Autodesk Inventor part; units mm, degrees
(part 2 of 2)
sketch "Sketch4" plane through (0, 2.3813, 0) normal (0, 1, 0) x (1, 0, 0)
  line L0 (28.188, 43.6739) -> (29.5096, 45.2433) construction
  spline S0 degree 3 poles (28.188, 43.6739) (29.5096, 45.2433) (31.9877, 45.6564) (33.3919, 45.6563) (35.0439, 45.6563) (37.3568, 44.8303) (37.3568, 41.6915) (37.3568, 40.122) (36.8611, 38.3874) (35.8699, 37.3136) knots 15 15 15 15 16 16 16 17 17 17 18 18 18 18
  line L1 (29.5096, 45.2433) -> (31.9877, 45.6564) construction
  line L2 (31.9877, 45.6564) -> (33.3919, 45.6563) construction
  line L3 (33.3919, 45.6563) -> (35.0439, 45.6563) construction
  line L4 (35.0439, 45.6563) -> (37.3568, 44.8303) construction
  line L5 (37.3568, 44.8303) -> (37.3568, 41.6915) construction
  line L6 (37.3568, 41.6915) -> (37.3568, 40.122) construction
  line L7 (37.3568, 40.122) -> (36.8611, 38.3874) construction
  line L8 (36.8611, 38.3874) -> (35.8699, 37.3136) construction
  spline S1 degree 3 poles (35.8699, 37.3136) (34.7135, 35.9094) (33.6397, 35.8268) (31.8224, 35.6616) (30.9138, 35.579) (30.8312, 35.579) (30.666, 35.579) (30.5834, 35.579) (30.253, 35.4964) (30.253, 35.0833) knots 18 18 18 18 19 19 19 20 20 20 21 21 21 21
  line L9 (35.8699, 37.3136) -> (34.7135, 35.9094) construction
  line L10 (34.7135, 35.9094) -> (33.6397, 35.8268) construction
  line L11 (33.6397, 35.8268) -> (31.8224, 35.6616) construction
  line L12 (31.8224, 35.6616) -> (30.9138, 35.579) construction
  line L13 (30.9138, 35.579) -> (30.8312, 35.579) construction
  line L14 (30.8312, 35.579) -> (30.666, 35.579) construction
  line L15 (30.666, 35.579) -> (30.5834, 35.579) construction
  line L16 (30.5834, 35.579) -> (30.253, 35.4964) construction
  line L17 (30.253, 35.4964) -> (30.253, 35.0833) construction
  spline S2 degree 3 poles (30.253, 35.0833) (30.253, 34.5877) (30.5834, 34.5877) (31.2442, 34.5877) knots 21 21 21 21 22 22 22 22
  line L18 (30.253, 35.0833) -> (30.253, 34.5877) construction
  line L19 (30.253, 34.5877) -> (30.5834, 34.5877) construction
  line L20 (30.5834, 34.5877) -> (31.2442, 34.5877) construction
  line L21 (31.2442, 34.5877) -> (33.2267, 34.5877)
  line L22 (13.0236, 12.4263) -> (20.0234, 12.4263)
  spline S3 degree 3 poles (20.0234, 12.4263) (20.3837, 12.4263) (20.8984, 12.4263) (20.8984, 12.9925) knots 1 1 1 1 2 2 2 2
  line L23 (20.0234, 12.4263) -> (20.3837, 12.4263) construction
  line L24 (20.3837, 12.4263) -> (20.8984, 12.4263) construction
  line L25 (20.8984, 12.4263) -> (20.8984, 12.9925) construction
  spline S4 degree 3 poles (20.8984, 12.9925) (20.8984, 13.5587) (20.3837, 13.5587) (20.0234, 13.5587) knots 2 2 2 2 3 3 3 3
  line L26 (20.8984, 12.9925) -> (20.8984, 13.5587) construction
  line L27 (20.8984, 13.5587) -> (20.3837, 13.5587) construction
  line L28 (20.3837, 13.5587) -> (20.0234, 13.5587) construction
  line L29 (20.0234, 13.5587) -> (13.0236, 13.5587)
  line L30 (13.0236, 13.5587) -> (13.0236, 20.4555)
  spline S5 degree 3 poles (13.0236, 20.4555) (13.0236, 20.8673) (13.0236, 21.4334) (12.4574, 21.4334) (11.8913, 21.4334) (11.8913, 20.9187) (11.8913, 20.5585) knots 5 5 5 5 6 6 6 7 7 7 7
  line L31 (13.0236, 20.4555) -> (13.0236, 20.8673) construction
  line L32 (13.0236, 20.8673) -> (13.0236, 21.4334) construction
  line L33 (13.0236, 21.4334) -> (12.4574, 21.4334) construction
  line L34 (12.4574, 21.4334) -> (11.8913, 21.4334) construction
  line L35 (11.8913, 21.4334) -> (11.8913, 20.9187) construction
  line L36 (11.8913, 20.9187) -> (11.8913, 20.5585) construction
  line L37 (11.8913, 20.5585) -> (11.8913, 13.5587)
  line L38 (11.8913, 13.5587) -> (4.8915, 13.5587)
  spline S6 degree 3 poles (4.8915, 13.5587) (4.5312, 13.5587) (3.965, 13.5587) (3.965, 12.9925) knots 9 9 9 9 10 10 10 10
  line L39 (4.8915, 13.5587) -> (4.5312, 13.5587) construction
  line L40 (4.5312, 13.5587) -> (3.965, 13.5587) construction
  line L41 (3.965, 13.5587) -> (3.965, 12.9925) construction
  spline S7 degree 3 poles (3.965, 12.9925) (3.965, 12.4264) (4.5312, 12.4264) (4.8915, 12.4263) knots 10 10 10 10 11 11 11 11
  line L42 (3.965, 12.9925) -> (3.965, 12.4264) construction
  line L43 (3.965, 12.4264) -> (4.5312, 12.4264) construction
  line L44 (4.5312, 12.4264) -> (4.8915, 12.4263) construction
  line L45 (4.8915, 12.4263) -> (11.8913, 12.4263)
  line L46 (11.8913, 12.4263) -> (11.8913, 5.6324)
  line L47 (11.8913, 5.6324) -> (4.8915, 5.6324)
  spline S8 degree 3 poles (4.8915, 5.6324) (4.5312, 5.6324) (3.965, 5.6324) (3.965, 5.0663) knots 14 14 14 14 15 15 15 15
  line L48 (4.8915, 5.6324) -> (4.5312, 5.6324) construction
  line L49 (4.5312, 5.6324) -> (3.965, 5.6324) construction
  line L50 (3.965, 5.6324) -> (3.965, 5.0663) construction
  spline S9 degree 3 poles (3.965, 5.0663) (3.965, 4.5001) (4.5312, 4.5001) (4.8915, 4.5001) knots 15 15 15 15 16 16 16 16
  line L51 (3.965, 5.0663) -> (3.965, 4.5001) construction
  line L52 (3.965, 4.5001) -> (4.5312, 4.5001) construction
  line L53 (4.5312, 4.5001) -> (4.8915, 4.5001) construction
  line L54 (4.8915, 4.5001) -> (20.0234, 4.5001)
  spline S10 degree 3 poles (20.0234, 4.5001) (20.3837, 4.5001) (20.8984, 4.5001) (20.8984, 5.0663) knots 17 17 17 17 18 18 18 18
  line L55 (20.0234, 4.5001) -> (20.3837, 4.5001) construction
  line L56 (20.3837, 4.5001) -> (20.8984, 4.5001) construction
  line L57 (20.8984, 4.5001) -> (20.8984, 5.0663) construction
  spline S11 degree 3 poles (20.8984, 5.0663) (20.8984, 5.6324) (20.3837, 5.6324) (20.0234, 5.6324) knots 18 18 18 18 19 19 19 19
  line L58 (20.8984, 5.0663) -> (20.8984, 5.6324) construction
  line L59 (20.8984, 5.6324) -> (20.3837, 5.6324) construction
  line L60 (20.3837, 5.6324) -> (20.0234, 5.6324) construction
  line L61 (20.0234, 5.6324) -> (13.0236, 5.6324)
  line L62 (13.0236, 5.6324) -> (13.0236, 12.4263)
  spline S12 degree 3 poles (33.2267, 34.5877) (36.1177, 34.5877) (38.1828, 32.6053) (38.1828, 28.6404) (38.1828, 24.0973) (35.4569, 22.6931) (33.3919, 22.6931) (31.905, 22.6931) (28.601, 23.1061) (27.1141, 25.3364) knots 0 0 0 0 1 1 1 2 2 2 3 3 3 3
  line L63 (33.2267, 34.5877) -> (36.1177, 34.5877) construction
  line L64 (36.1177, 34.5877) -> (38.1828, 32.6053) construction
  line L65 (38.1828, 32.6053) -> (38.1828, 28.6404) construction
  line L66 (38.1828, 28.6404) -> (38.1828, 24.0973) construction
  line L67 (38.1828, 24.0973) -> (35.4569, 22.6931) construction
  line L68 (35.4569, 22.6931) -> (33.3919, 22.6931) construction
  line L69 (33.3919, 22.6931) -> (31.905, 22.6931) construction
  line L70 (31.905, 22.6931) -> (28.601, 23.1061) construction
  line L71 (28.601, 23.1061) -> (27.1141, 25.3364) construction
  spline S13 degree 3 poles (27.1141, 25.3364) (28.8488, 25.3364) (29.2618, 26.5754) (29.2618, 27.4014) (29.2618, 28.5578) (28.3532, 29.3838) (27.1968, 29.3838) (26.2055, 29.3838) (25.1317, 28.723) (25.1317, 27.2362) (25.1317, 23.7669) (28.9314, 21.5367) (33.3919, 21.5367) (38.5132, 21.5367) (42.065, 25.0059) (42.065, 28.6404) (42.065, 31.5315) (39.7522, 34.4225) (35.7047, 35.2485) knots 3 3 3 3 4 4 4 5 5 5 6 6 6 7 7 7 8 8 8 9 9 9 9
  line L72 (27.1141, 25.3364) -> (28.8488, 25.3364) construction
  line L73 (28.8488, 25.3364) -> (29.2618, 26.5754) construction
  line L74 (29.2618, 26.5754) -> (29.2618, 27.4014) construction
  line L75 (29.2618, 27.4014) -> (29.2618, 28.5578) construction
  line L76 (29.2618, 28.5578) -> (28.3532, 29.3838) construction
  line L77 (28.3532, 29.3838) -> (27.1968, 29.3838) construction
  line L78 (27.1968, 29.3838) -> (26.2055, 29.3838) construction
  line L79 (26.2055, 29.3838) -> (25.1317, 28.723) construction
  line L80 (25.1317, 28.723) -> (25.1317, 27.2362) construction
  line L81 (25.1317, 27.2362) -> (25.1317, 23.7669) construction
  line L82 (25.1317, 23.7669) -> (28.9314, 21.5367) construction
  line L83 (28.9314, 21.5367) -> (33.3919, 21.5367) construction
  line L84 (33.3919, 21.5367) -> (38.5132, 21.5367) construction
  line L85 (38.5132, 21.5367) -> (42.065, 25.0059) construction
  line L86 (42.065, 25.0059) -> (42.065, 28.6404) construction
  line L87 (42.065, 28.6404) -> (42.065, 31.5315) construction
  line L88 (42.065, 31.5315) -> (39.7522, 34.4225) construction
  line L89 (39.7522, 34.4225) -> (35.7047, 35.2485) construction
  spline S14 degree 3 poles (35.7047, 35.2485) (39.5044, 36.6528) (40.9086, 39.3786) (40.9086, 41.6915) (40.9086, 44.5825) (37.6046, 46.7302) (33.4745, 46.7302) (29.427, 46.7302) (26.2881, 44.7477) (26.2881, 41.7741) (26.2881, 40.5351) (27.1142, 39.8742) (28.188, 39.8742) (29.3444, 39.8742) (30.0878, 40.7003) (30.0878, 41.6915) (30.0878, 42.7653) (29.3444, 43.5913) (28.188, 43.6739) knots 9 9 9 9 10 10 10 11 11 11 12 12 12 13 13 13 14 14 14 15 15 15 15
  line L90 (35.7047, 35.2485) -> (39.5044, 36.6528) construction
  line L91 (39.5044, 36.6528) -> (40.9086, 39.3786) construction
  line L92 (40.9086, 39.3786) -> (40.9086, 41.6915) construction
  line L93 (40.9086, 41.6915) -> (40.9086, 44.5825) construction
  line L94 (40.9086, 44.5825) -> (37.6046, 46.7302) construction
  line L95 (37.6046, 46.7302) -> (33.4745, 46.7302) construction
  line L96 (33.4745, 46.7302) -> (29.427, 46.7302) construction
  line L97 (29.427, 46.7302) -> (26.2881, 44.7477) construction
  line L98 (26.2881, 44.7477) -> (26.2881, 41.7741) construction
  line L99 (26.2881, 41.7741) -> (26.2881, 40.5351) construction
  line L100 (26.2881, 40.5351) -> (27.1142, 39.8742) construction
  line L101 (27.1142, 39.8742) -> (28.188, 39.8742) construction
  line L102 (28.188, 39.8742) -> (29.3444, 39.8742) construction
  line L103 (29.3444, 39.8742) -> (30.0878, 40.7003) construction
  line L104 (30.0878, 40.7003) -> (30.0878, 41.6915) construction
  line L105 (30.0878, 41.6915) -> (30.0878, 42.7653) construction
  line L106 (30.0878, 42.7653) -> (29.3444, 43.5913) construction
  line L107 (29.3444, 43.5913) -> (28.188, 43.6739) construction
  line L108 (25.1359, -42.0708) -> (-42.6059, -42.0708)
  line L109 (-42.6059, -42.0708) -> (-42.6059, 25.671)
  line L110 (-42.6059, 25.671) -> (17.5159, 25.671)
  spline S15 degree 3 poles (17.5159, 25.671) (20.4794, 22.7075) (22.1725, 21.0145) (25.1359, 18.051) knots 3 3 3 3 4 4 4 4
  line L111 (17.5159, 25.671) -> (20.4794, 22.7075) construction
  line L112 (20.4794, 22.7075) -> (22.1725, 21.0145) construction
  line L113 (22.1725, 21.0145) -> (25.1359, 18.051) construction
  line L114 (25.1359, 18.051) -> (25.1359, -42.0708)
  spline S16 degree 3 poles (-17.3729, 2.4446) (-16.9814, 3.7171) (-16.3941, 6.1641) (-16.3941, 6.4577) knots 0 0 0 0 1 1 1 1
  line L115 (-17.3729, 2.4446) -> (-16.9814, 3.7171) construction
  line L116 (-16.9814, 3.7171) -> (-16.3941, 6.1641) construction
  line L117 (-16.3941, 6.1641) -> (-16.3941, 6.4577) construction
  spline S17 degree 3 poles (-16.3941, 6.4577) (-16.3941, 7.5344) (-17.1772, 8.1217) (-18.2539, 8.1217) knots 1 1 1 1 2 2 2 2
  line L118 (-16.3941, 6.4577) -> (-16.3941, 7.5344) construction
  line L119 (-16.3941, 7.5344) -> (-17.1772, 8.1217) construction
  line L120 (-17.1772, 8.1217) -> (-18.2539, 8.1217) construction
  spline S18 degree 3 poles (-18.2539, 8.1217) (-18.3517, 8.1217) (-20.1136, 8.0238) (-20.7009, 5.8705) knots 2 2 2 2 3 3 3 3
  line L121 (-18.2539, 8.1217) -> (-18.3517, 8.1217) construction
  line L122 (-18.3517, 8.1217) -> (-20.1136, 8.0238) construction
  line L123 (-20.1136, 8.0238) -> (-20.7009, 5.8705) construction
  line L124 (-20.7009, 5.8705) -> (-29.7059, -30.2475)
  spline S19 degree 3 poles (-29.7059, -30.2475) (-29.9017, -31.0305) (-29.9017, -31.1284) (-29.9017, -31.3241) knots 4 4 4 4 5 5 5 5
  line L125 (-29.7059, -30.2475) -> (-29.9017, -31.0305) construction
  line L126 (-29.9017, -31.0305) -> (-29.9017, -31.1284) construction
  line L127 (-29.9017, -31.1284) -> (-29.9017, -31.3241) construction
  spline S20 degree 3 poles (-29.9017, -31.3241) (-29.9017, -32.2051) (-29.2165, -32.9881) (-28.1398, -32.9881) (-26.8674, -32.9881) (-26.0843, -31.8136) (-25.9864, -31.6178) knots 5 5 5 5 6 6 6 7 7 7 7
  line L128 (-29.9017, -31.3241) -> (-29.9017, -32.2051) construction
  line L129 (-29.9017, -32.2051) -> (-29.2165, -32.9881) construction
  line L130 (-29.2165, -32.9881) -> (-28.1398, -32.9881) construction
  line L131 (-28.1398, -32.9881) -> (-26.8674, -32.9881) construction
  line L132 (-26.8674, -32.9881) -> (-26.0843, -31.8136) construction
  line L133 (-26.0843, -31.8136) -> (-25.9864, -31.6178) construction
  spline S21 degree 3 poles (-25.9864, -31.6178) (-25.6928, -31.1284) (-24.9098, -27.8004) (-22.5606, -18.2082) knots 7 7 7 7 8 8 8 8
  line L134 (-25.9864, -31.6178) -> (-25.6928, -31.1284) construction
  line L135 (-25.6928, -31.1284) -> (-24.9098, -27.8004) construction
  line L136 (-24.9098, -27.8004) -> (-22.5606, -18.2082) construction
  spline S22 degree 3 poles (-22.5606, -18.2082) (-20.5051, -19.8721) (-17.6666, -20.1658) (-16.492, -20.1658) (-12.0874, -20.1658) (-9.6404, -17.3272) (-8.1722, -15.5654) knots 8 8 8 8 9 9 9 10 10 10 10
  line L137 (-22.5606, -18.2082) -> (-20.5051, -19.8721) construction
  line L138 (-20.5051, -19.8721) -> (-17.6666, -20.1658) construction
  line L139 (-17.6666, -20.1658) -> (-16.492, -20.1658) construction
  line L140 (-16.492, -20.1658) -> (-12.0874, -20.1658) construction
  line L141 (-12.0874, -20.1658) -> (-9.6404, -17.3272) construction
  line L142 (-9.6404, -17.3272) -> (-8.1722, -15.5654) construction
  spline S23 degree 3 poles (-8.1722, -15.5654) (-7.5849, -18.4039) (-5.2358, -20.1658) (-2.4951, -20.1658) (-0.3417, -20.1658) (1.1265, -18.6976) (2.1053, -16.74) knots 10 10 10 10 11 11 11 12 12 12 12
  line L143 (-8.1722, -15.5654) -> (-7.5849, -18.4039) construction
  line L144 (-7.5849, -18.4039) -> (-5.2358, -20.1658) construction
  line L145 (-5.2358, -20.1658) -> (-2.4951, -20.1658) construction
  line L146 (-2.4951, -20.1658) -> (-0.3417, -20.1658) construction
  line L147 (-0.3417, -20.1658) -> (1.1265, -18.6976) construction
  line L148 (1.1265, -18.6976) -> (2.1053, -16.74) construction
  spline S24 degree 3 poles (2.1053, -16.74) (3.182, -14.4887) (3.965, -10.6714) (3.965, -10.5735) knots 12 12 12 12 13 13 13 13
  line L149 (2.1053, -16.74) -> (3.182, -14.4887) construction
  line L150 (3.182, -14.4887) -> (3.965, -10.6714) construction
  line L151 (3.965, -10.6714) -> (3.965, -10.5735) construction
  spline S25 degree 3 poles (3.965, -10.5735) (3.965, -9.8883) (3.3777, -9.8883) (3.182, -9.8883) (2.5947, -9.8883) (2.4968, -10.182) (2.301, -11.0629) knots 13 13 13 13 14 14 14 15 15 15 15
  line L152 (3.965, -10.5735) -> (3.965, -9.8883) construction
  line L153 (3.965, -9.8883) -> (3.3777, -9.8883) construction
  line L154 (3.3777, -9.8883) -> (3.182, -9.8883) construction
  line L155 (3.182, -9.8883) -> (2.5947, -9.8883) construction
  line L156 (2.5947, -9.8883) -> (2.4968, -10.182) construction
  line L157 (2.4968, -10.182) -> (2.301, -11.0629) construction
  spline S26 degree 3 poles (2.301, -11.0629) (1.3222, -15.076) (0.1477, -18.7955) (-2.3972, -18.7955) (-4.0612, -18.7955) (-4.257, -17.1315) (-4.257, -15.9569) (-4.257, -14.5866) (-3.5718, -11.6502) (-3.0824, -9.3989) knots 15 15 15 15 16 16 16 17 17 17 18 18 18 18
  line L158 (2.301, -11.0629) -> (1.3222, -15.076) construction
  line L159 (1.3222, -15.076) -> (0.1477, -18.7955) construction
  line L160 (0.1477, -18.7955) -> (-2.3972, -18.7955) construction
  line L161 (-2.3972, -18.7955) -> (-4.0612, -18.7955) construction
  line L162 (-4.0612, -18.7955) -> (-4.257, -17.1315) construction
  line L163 (-4.257, -17.1315) -> (-4.257, -15.9569) construction
  line L164 (-4.257, -15.9569) -> (-4.257, -14.5866) construction
  line L165 (-4.257, -14.5866) -> (-3.5718, -11.6502) construction
  line L166 (-3.5718, -11.6502) -> (-3.0824, -9.3989) construction
  line L167 (-3.0824, -9.3989) -> (-1.3205, -2.6452)
  spline S27 degree 3 poles (-1.3205, -2.6452) (-1.1248, -1.7642) (-0.4396, 0.5849) (-0.2438, 1.5637) (0.0498, 3.0319) (0.735, 5.381) (0.735, 5.7726) knots 19 19 19 19 20 20 20 21 21 21 21
  line L168 (-1.3205, -2.6452) -> (-1.1248, -1.7642) construction
  line L169 (-1.1248, -1.7642) -> (-0.4396, 0.5849) construction
  line L170 (-0.4396, 0.5849) -> (-0.2438, 1.5637) construction
  line L171 (-0.2438, 1.5637) -> (0.0498, 3.0319) construction
  line L172 (0.0498, 3.0319) -> (0.735, 5.381) construction
  line L173 (0.735, 5.381) -> (0.735, 5.7726) construction
  spline S28 degree 3 poles (0.735, 5.7726) (0.735, 6.8492) (-0.146, 7.4365) (-1.1248, 7.4365) (-1.4184, 7.4365) (-3.0824, 7.3386) (-3.5718, 5.2832) knots 21 21 21 21 22 22 22 23 23 23 23
  line L174 (0.735, 5.7726) -> (0.735, 6.8492) construction
  line L175 (0.735, 6.8492) -> (-0.146, 7.4365) construction
  line L176 (-0.146, 7.4365) -> (-1.1248, 7.4365) construction
  line L177 (-1.1248, 7.4365) -> (-1.4184, 7.4365) construction
  line L178 (-1.4184, 7.4365) -> (-3.0824, 7.3386) construction
  line L179 (-3.0824, 7.3386) -> (-3.5718, 5.2832) construction
  line L180 (-3.5718, 5.2832) -> (-6.5082, -6.4625)
  spline S29 degree 3 poles (-6.5082, -6.4625) (-7.1934, -9.5947) (-7.8785, -12.1396) (-8.0743, -12.8247) knots 24 24 24 24 25 25 25 25
  line L181 (-6.5082, -6.4625) -> (-7.1934, -9.5947) construction
  line L182 (-7.1934, -9.5947) -> (-7.8785, -12.1396) construction
  line L183 (-7.8785, -12.1396) -> (-8.0743, -12.8247) construction
  spline S30 degree 3 poles (-8.0743, -12.8247) (-8.1722, -13.1184) (-11.1086, -18.7954) (-16.1984, -18.7954) (-19.3306, -18.7954) (-20.7988, -16.74) (-20.7988, -13.3141) (-20.7988, -11.5523) (-20.4072, -9.7904) (-19.9178, -8.0286) knots 25 25 25 25 26 26 26 27 27 27 28 28 28 28
  line L184 (-8.0743, -12.8247) -> (-8.1722, -13.1184) construction
  line L185 (-8.1722, -13.1184) -> (-11.1086, -18.7954) construction
  line L186 (-11.1086, -18.7954) -> (-16.1984, -18.7954) construction
  line L187 (-16.1984, -18.7954) -> (-19.3306, -18.7954) construction
  line L188 (-19.3306, -18.7954) -> (-20.7988, -16.74) construction
  line L189 (-20.7988, -16.74) -> (-20.7988, -13.3141) construction
  line L190 (-20.7988, -13.3141) -> (-20.7988, -11.5523) construction
  line L191 (-20.7988, -11.5523) -> (-20.4072, -9.7904) construction
  line L192 (-20.4072, -9.7904) -> (-19.9178, -8.0286) construction
  line L193 (-19.9178, -8.0286) -> (-17.3729, 2.4446)
  point P0 (0, 0)
  constraints: 40 end point, 93 other
extrude "Extrusion3" cut sketch "Sketch4" against normal blind 0.25
equation "\"d7\" = suppourtPanelThickness"
equation "\"d28\" = d27"
equation "\"panelChamfer\" = 75"
equation "\"suppourtPanelThickness\" = 2.38125"
body "Solid1"
